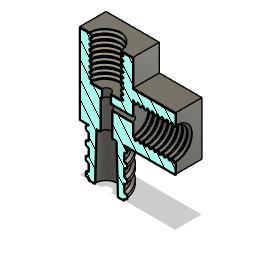
SYRSEP_V1 (Autodesk Fusion 360 design; units mm, degrees)
Autodesk Fusion 360 part; units mm, degrees
sketch "Sketch1" plane through (0, 0, 0) normal (0, 1, 0) x (1, 0, 0)
  line L0 (5, -5) -> (-5, -5)
  line L1 (-5, -5) -> (-5, 5)
  line L2 (-5, 5) -> (5, 5)
  line L3 (5, 5) -> (5, -5)
  line L4 (5, -5) -> (-5, 5) construction
  line L5 (-5, -5) -> (5, 5) construction
  dimension "d1" = 10
  dimension "d2" = 10
  constraint horizontal L0
  constraint perpendicular L0 L1
  constraint parallel L0 L2
  constraint parallel L1 L3
  constraint coincident L4 origin
  constraint coincident L5 origin
  measures "d1" distance of L0.end L1.end
  measures "d2" distance of L1.end L2.end
extrude "Extrude1" add sketch "Sketch1" along normal blind 15
hole "Hole1" at (0, 15, 0) direction (0, -1, 0) diameter 5.474 depth 8 tip angle 180
thread "Thread1" "ANSI Unified Screw Threads 0.25 1/4-28 UNF 1B" major diameter 6.35 minor diameter 5.4737 pitch 0.9071 angle 60 modelled right hand crest width 0.2395 on face at (0.1364, 12.3333, 2.7336) crest through (0, 14.7732, 2.7368)
sketch "Sketch3" plane through (0, 0, 0) normal (0, -1, 0) x (-1, 0, 0)
  circle A0 centre (0, 0) radius 3.35
  circle A1 centre (0, 0) radius 1.8795
  arc A2 (-1.24, 3.695) -> (-3.4072, 1.8925) centre (0, 0) ccw
  arc A3 (0.004, 3.3446) -> (-1.24, 3.695) centre (-1.487, 0.435) ccw
  arc A4 (-3.4072, 1.8925) -> (-3.2921, 0.6045) centre (-0.156, 1.534) ccw
  arc A5 (1.24, -3.695) -> (3.4072, -1.8925) centre (0, 0) ccw
  arc A6 (-0.004, -3.3446) -> (1.24, -3.695) centre (1.487, -0.435) ccw
  arc A7 (3.4072, -1.8925) -> (3.2921, -0.6045) centre (0.156, -1.534) ccw
  line L0 (0, 0, 0) -> (0, 0, 9)
extrude "Extrude2" add sketch "Sketch3" along normal blind 9 contours A0
extrude "Extrude3" cut sketch "Sketch3" along normal blind 9 draft 1.72 contours A1
sweep "Sweep1" add twist angle 648 profiles "Sketch3" path "Sketch3" along L0 section 1 contours A0 A2 A3 A4 | A0 A5 A6 A7
hole "Hole2" at (0, 0, 0) direction (0, 1, 0) diameter 2.2 depth 5.5 tip angle 180
hole "Hole3" at (0, 0, 0) direction (0, 1, 0) diameter 1.7 end through all
sketch "Sketch4" plane through (5, 0, 0) normal (1, 0, 0) x (0, 0, -1)
  line L0 (-5, 0) -> (5, 0)
  line L1 (5, 0) -> (5, 15)
  line L2 (5, 15) -> (-5, 15)
  line L3 (-5, 15) -> (-5, 0)
  line L4 (5, 0) -> (-5, 0)
  line L5 (-5, 0) -> (-5, 10)
  line L6 (-5, 10) -> (5, 10)
  line L7 (5, 10) -> (5, 0)
  line L8 (-5, 10) -> (5, 0) construction
  line L9 (-5, 0) -> (5, 10) construction
  dimension "d25" = 10
  constraint horizontal L4
  constraint vertical L5
  constraint horizontal L6
  constraint vertical L7
  constraint coincident L3 L5.end
  constraint coincident L0.end L1.start
  measures "d25" distance of L0.end L6.end
extrude "Extrude4" add sketch "Sketch4" along normal blind 8 contours L0 L1 L3 L4 L5 L6 L7
hole "Hole4" at (13, 5, 0) direction (-1, 0, 0) diameter 5.474 depth 8 tip angle 180
thread "Thread2" "ANSI Unified Screw Threads 0.25 1/4-28 UNF 1B" major diameter 6.35 minor diameter 5.4737 pitch 0.9071 angle 60 modelled right hand crest width 0.2395 on face at (10.3333, 5.2725, -2.7234) crest through (12.7732, 7.7369, 0)
hole "Hole5" at (5, 5, 0) direction (-1, 0, 0) diameter 1 depth 5 tip angle 180
